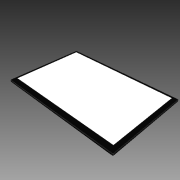
# Autodesk Inventor part: main_lcd_panel
Saved by Autodesk Inventor 2014 (Build 180170000, 170)
## iProperties
Created: 2014-03-22
Part Number: main_lcd_panel
Material: Generic
Document SubType Name: Modeling
Designer: buben
Density: 1 g/cm^3
Appearance: Anodized - Black
Author: buben
Autodesk Inventor part; units mm, degrees
ref_plane "YZ Plane" through (0, 0, 0) normal (1, 0, 0) x (0, 1, 0)
ref_plane "XZ Plane" through (0, 0, 0) normal (0, 1, 0) x (-1, 0, 0)
ref_plane "XY Plane" through (0, 0, 0) normal (0, 0, 1) x (1, 0, 0)
sketch "Sketch1" plane through (0, 0, 0) normal (0, 1, 0) x (-1, 0, 0)
  line L0 (0, 0) -> (-161.5, 0)
  line L1 (-161.5, 0) -> (-161.5, -107)
  line L2 (-161.5, -107) -> (0, -107)
  line L3 (0, -107) -> (0, 0)
  dimension "d0" = 161.5
  dimension "d1" = 107
  constraints: 8 end point, 2 parallel, 1 horizontal, 1 perpendicular
  measures "d0" distance of L0.start L0.end
  measures "d1" distance of L2.end L0.start
extrude "Extrusion1" add sketch "Sketch1" along normal blind 2.5
sketch "Sketch2" plane through (0, 2.5, 0) normal (0, 1, 0) x (1, 0, 0)
  line L0 (161.5, 107) -> (0, 107) projected
  line L1 (0, 107) -> (0, 0) projected
  line L2 (3, 104) -> (155, 104)
  line L3 (155, 104) -> (155, 8)
  line L4 (155, 8) -> (3, 8)
  line L5 (3, 8) -> (3, 104)
  dimension "d4" = 3
  dimension "d5" = 3
  dimension "d6" = 152
  dimension "d7" = 96
  constraints: 8 end point, 2 parallel, 1 horizontal, 1 perpendicular
  measures "d4" distance between parallel lines of L5 L1
  measures "d5" distance between parallel lines of L0 L2
  measures "d6" distance of L3.end L4.end
  measures "d7" distance of L2.end L3.end
extrude "Extrusion2" cut sketch "Sketch2" against normal blind 0.1
fillet "Fillet1" radius 0.4 8 edges at (0, 2.5, -53.5) (80.75, 2.5, -107) (80.75, 2.5, 0) (161.5, 2.5, -53.5) (80.75, 0, 0) (0, 0, -53.5) (80.75, 0, -107) (161.5, 0, -53.5)
fillet "Fillet2" radius 1.2 12 edges at (161.3828, 2.3828, -0.1172) (161.3828, 0.1172, -0.1172) (161.5, 1.25, 0) (0.1172, 2.3828, -0.1172) (0.1172, 0.1172, -0.1172) (0, 1.25, 0) (0.1172, 2.3828, -106.8828) (0.1172, 0.1172, -106.8828) (0, 1.25, -107) (161.3828, 2.3828, -106.8828) (161.3828, 0.1172, -106.8828) (161.5, 1.25, -107)
body "Solid1"
